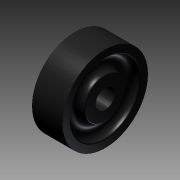
# Autodesk Inventor part: bane bots wheel hub 3 in
Saved by Autodesk Inventor 2012 (Build 160160000, 160)
## iProperties
Created: 2013-07-13
Part Number: bane bots wheel hub 3 in
Material: Default
Document SubType Name: Modeling
Designer: Bryce
Density: 1 g/cm^3
Author: Bryce
Autodesk Inventor part; units mm, degrees
ref_plane "YZ Plane" through (0, 0, 0) normal (1, 0, 0) x (0, 1, 0)
ref_plane "XZ Plane" through (0, 0, 0) normal (0, 1, 0) x (-1, 0, 0)
ref_plane "XY Plane" through (0, 0, 0) normal (0, 0, 1) x (1, 0, 0)
sketch "Sketch1" plane through (0, 0, 0) normal (0, 0, 1) x (1, 0, 0)
  line L0 (0, 0) -> (20.32, 0)
  line L1 (20.32, 0) -> (20.32, 7.3025)
  line L2 (20.32, 22.225) -> (0, 22.225)
  line L3 (0, 22.225) -> (0, 16.8275)
  line L4 (0, -6.35) -> (20.32, -6.35) construction
  arc A0 (0, 7.3025) -> (0, 16.8275) centre (0, 12.065) ccw
  arc A1 (20.32, 16.8275) -> (20.32, 7.3025) centre (20.32, 12.065) ccw
  line L5 (0, 16.8275) -> (0, 7.3025) construction
  line L6 (0, 7.3025) -> (0, 0)
  line L7 (20.32, 16.8275) -> (20.32, 22.225)
  line L8 (20.32, 7.3025) -> (20.32, 16.8275) construction
  dimension "d0" = 20.32
  dimension "d1" = 22.225
  dimension "d3" = 6.35
  dimension "d4" = 10.16
  dimension "d5" = 4.7625
  dimension "d6" = 4.7625
  dimension "d7" = 10.16
  constraints: 18 end point, 10 parallel, 6 perpendicular, 4 point on circle, 2 centre point, 2 midpoint, 2 point on line, 1 horizontal, 1 vertical alignment
  measures "d0" distance of L0.start L0.end
  measures "d1" distance of L2.end L0.start
  measures "d3" distance between parallel lines of L4 L0
  measures "d4" distance from line of L2 A0.centre
  measures "d5" radius of A0
  measures "d6" radius of A1
  measures "d7" distance from line of L2 A1.centre
revolve "Revolution1" add sketch "Sketch1" angle 360 about axis through (0, -6.35, 0) along (1, 0, 0)
fillet "Fillet1" radius 0.7937 4 edges at (20.32, -29.5275, 0) (20.32, -20.0025, 0) (0, -20.0025, 0) (0, -29.5275, 0)
equation "\"d6\" = d5"
equation "\"d7\" = d4"
body "Solid1"
